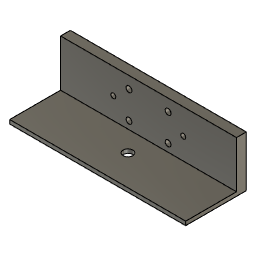
simple mount 2 v2 (Autodesk Fusion 360 design; units mm, degrees)
Autodesk Fusion 360 part; units mm, degrees
sketch "Sketch1" plane through (0, 0, 0) normal (0, 1, 0) x (1, 0, 0)
  line L0 (0, 0) -> (90, 0)
  line L1 (90, 0) -> (90, -26)
  line L2 (0, 0) -> (0, -26)
  line L3 (0, -26) -> (90, -26)
  dimension "d1" = 90
  dimension "d2" = 26
  dimension "d3" = 26
  constraint coincident L0.start L2.start
  constraint horizontal L0
  constraint perpendicular L0 L1
  constraint perpendicular L0 L2
  measures "d1" distance of L0.start L0.end
  measures "d2" distance of L0.end L1.end
  measures "d3" distance of L0.start L2.end
extrude "Extrude1" add sketch "Sketch1" along normal blind 5
sketch "Sketch2" plane through (0, 0, 0) normal (0, -1, 0) x (1, 0, 0)
  line L0 (0, 26) -> (0, 0)
  line L1 (0, 0) -> (90, 0)
  line L2 (90, 0) -> (90, 26)
  line L3 (90, 26) -> (0, 26)
  line L4 (0, 0) -> (90, 0)
  line L5 (90, 0) -> (90, 2)
  line L6 (0, 0) -> (0, 2)
  line L7 (0, 2) -> (90, 2)
  dimension "d6" = 2
  dimension "d7" = 2
  constraint coincident L0.end L1.start
  constraint coincident L1.end L2.start
  constraint perpendicular L1 L5
  constraint perpendicular L1 L6
  measures "d6" distance of L1.end L5.end
  measures "d7" distance of L0.end L6.end
extrude "Extrude2" add sketch "Sketch2" along normal blind 26 contours L0 L1 L2 L4 L5 L6 L7
sketch "Sketch3" plane through (0, 0, 0) normal (0, 0, -1) x (1, 0, 0)
  line L0 (0, 26) -> (0, -5)
  line L1 (0, -5) -> (90, -5)
  line L2 (90, -5) -> (90, 26)
  line L3 (90, 26) -> (0, 26)
  line L4 (90, 10.5) -> (0, 10.5) construction
  line L5 (45, 26) -> (45, -5) construction
  circle A0 centre (45, 10.5) radius 2.5
  dimension "d10" = 5
  constraint midpoint L2 L4.start
  constraint midpoint L0 L4.end
  constraint midpoint L3 L5.start
  constraint perpendicular L4 L5
  constraint midpoint L4 A0.centre
  measures "d10" diameter of A0
extrude "Extrude3" cut sketch "Sketch3" against normal blind 3 contours A0
sketch "Sketch4" plane through (0, 5, 0) normal (0, 1, 0) x (-1, 0, 0)
  line L0 (0, 0) -> (0, 26)
  line L1 (0, 26) -> (-90, 26)
  line L2 (-90, 26) -> (-90, 0)
  line L3 (-90, 0) -> (0, 0)
  line L4 (-90, 13) -> (0, 13) construction
  line L5 (-45, 26) -> (-45, 0) construction
  line L6 (-90, 7.6084) -> (-73, 7.6084) construction
  line L7 (-73, 7.6084) -> (-71.75, 7.6084) construction
  line L8 (-70.5, 7.6084) -> (-28.5, 7.6084) construction
  line L9 (-28.5, 7.6084) -> (-27.25, 7.6084) construction
  line L10 (-27.25, 7.6084) -> (-27.25, 13) construction
  line L11 (-71.75, 7.6084) -> (-71.75, 13) construction
  circle A0 centre (-27.25, 13) radius 1.25
  circle A1 centre (-71.75, 13) radius 1.25
  dimension "d13" = 17
  dimension "d15" = 1.25
  dimension "d17" = 42
  dimension "d18" = 1.25
  dimension "d20" = 2.5
  dimension "d21" = 2.5
  constraint midpoint L2 L4.start
  constraint midpoint L0 L4.end
  constraint midpoint L1 L5.start
  constraint midpoint L3 L5.end
  constraint coincident L2 L6.start
  constraint perpendicular L2 L6
  constraint perpendicular L5 L7
  constraint parallel L7 L8
  constraint parallel L8 L9
  constraint coincident L4 L10.end
  constraint perpendicular L4 L10
  constraint coincident L4 L11.end
  constraint perpendicular L4 L11
  constraint coincident L10.end A0.centre
  constraint coincident L11.end A1.centre
  measures "d13" distance of L6.start L6.end
  measures "d15" distance of L6.end L7.end
  measures "d17" distance of L8.start L8.end
  measures "d18" distance of L8.end L9.end
  measures "d20" diameter of A0
  measures "d21" diameter of A1
sketch "Sketch5" plane through (0, 5, 0) normal (0, 1, 0) x (-1, 0, 0)
  line L0 (0, 0) -> (0, 26)
  line L1 (0, 26) -> (-90, 26)
  line L2 (-90, 26) -> (-90, 0)
  line L3 (-90, 0) -> (0, 0)
  line L4 (-90, 13) -> (0, 13) construction
  line L5 (-45, 0) -> (-45, 26) construction
  line L6 (-90, 19.9402) -> (0, 19.9402) construction
  line L7 (-35.0017, 26) -> (-35.0017, 0) construction
  line L8 (-54.9997, 26) -> (-54.9997, 0) construction
  circle A0 centre (-54.9997, 19.9402) radius 1.5
  circle A1 centre (-35.0017, 19.9402) radius 1.5
  line L9 (0, 6) -> (-90, 6) construction
  circle A2 centre (-35.0017, 6) radius 1.5
  circle A3 centre (-54.9997, 6) radius 1.5
  line L10 (-90, 13) -> (-62.75, 13) construction
  circle A4 centre (-62.75, 13) radius 1.25
  dimension "d24" = 3
  dimension "d25" = 3
  dimension "d27" = 3
  dimension "d28" = 3
  dimension "d29" = 27.25
  dimension "d30" = 2.5
  constraint midpoint L2 L4.start
  constraint midpoint L0 L4.end
  constraint midpoint L3 L5.start
  constraint midpoint L1 L5.end
  constraint coincident L2 L6.start
  constraint perpendicular L5 L6
  constraint coincident L1 L7.start
  constraint coincident L3 L7.end
  constraint perpendicular L3 L7
  constraint coincident L1 L8.start
  constraint coincident L3 L8.end
  constraint perpendicular L3 L8
  constraint coincident L8 A0.centre
  constraint coincident L6 A0.centre
  constraint coincident L6 A1.centre
  constraint coincident L7 A1.centre
  constraint coincident L0 L9.start
  constraint coincident L2 L9.end
  constraint perpendicular L2 L9
  constraint coincident L9 A2.centre
  constraint coincident L7 A2.centre
  constraint coincident L9 A3.centre
  constraint coincident L8 A3.centre
  constraint perpendicular L2 L10
  constraint coincident L10.end A4.centre
  measures "d24" diameter of A0
  measures "d25" diameter of A1
  measures "d27" diameter of A2
  measures "d28" diameter of A3
  measures "d29" distance of L4.start L10.end
  measures "d30" diameter of A4
extrude "Extrude5" cut sketch "Sketch5" against normal blind 5 contours A0 | A1 | A2 | A3 | A4
sketch "Sketch6" plane through (0, 5, 0) normal (0, 1, 0) x (-1, 0, 0)
  circle A0 centre (-54.9997, 19.9402) radius 1.5
  circle A1 centre (-54.9997, 6) radius 1.5
  circle A2 centre (-35.0017, 19.9402) radius 1.5
  circle A3 centre (-62.75, 13) radius 1.25
  circle A4 centre (-35.0017, 6) radius 1.5
  line L0 (0, 0) -> (0, 26)
  line L1 (0, 26) -> (-90, 26)
  line L2 (-90, 26) -> (-90, 0)
  line L3 (-90, 0) -> (0, 0)
  line L4 (0, 13) -> (-90, 13) construction
  line L5 (0, 9) -> (-27, 9) construction
  line L6 (-27, 9) -> (-27, 13) construction
  circle A5 centre (-27, 13) radius 1.25
  dimension "d33" = 27
  dimension "d34" = 2.5
  constraint midpoint L0 L4.start
  constraint perpendicular L0 L4
  constraint coincident L0 L5.start
  constraint perpendicular L0 L5
  constraint coincident L4 L6.end
  constraint perpendicular L4 L6
  constraint coincident L6.end A5.centre
  measures "d33" distance of L5.start L5.end
  measures "d34" diameter of A5
extrude "Extrude6" cut sketch "Sketch6" against normal blind 5 contours A5
